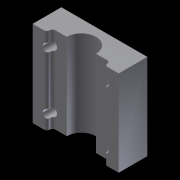
# Autodesk Inventor part: poleHolderA
Saved by Autodesk Inventor 2011 (Build 150239000, 239)
## iProperties
Created: 2012-10-15
Part Number: poleHolderA
Document SubType Name: Modeling
Designer: JohnHenry
Density: 1 g/cm^3
Author: JohnHenry
Autodesk Inventor part; units mm, degrees
ref_plane "YZ Plane" through (0, 0, 0) normal (1, 0, 0) x (0, 1, 0)
ref_plane "XZ Plane" through (0, 0, 0) normal (0, 1, 0) x (-1, 0, 0)
ref_plane "XY Plane" through (0, 0, 0) normal (0, 0, 1) x (1, 0, 0)
sketch "スケッチ1" plane through (0, 0, 0) normal (0, 0, 1) x (1, 0, 0)
  arc A0 (-5.1, 0) -> (5.1, 0) centre (0, 0) ccw
  line L0 (-15, 8) -> (15, 8)
  line L1 (15, 8) -> (15, 0)
  line L2 (15, 0) -> (5.1, 0)
  line L3 (-15, 0) -> (-15, 8)
  arc A1 (5.1, 0) -> (-5.1, 0) centre (0, 0) ccw
  line L4 (5.1, 0) -> (-5.1, 0)
  line L5 (-5.1, 0) -> (-15, 0)
  dimension "d0" = 10.2
  dimension "d1" = 30
  dimension "d2" = 15
  dimension "d3" = 8
  dimension "d4" = 0
  constraints: 12 end point, 4 parallel, 4 point on circle, 2 centre point, 1 coincident, 1 horizontal, 1 perpendicular, 1 point on line
  measures "d0" diameter of A0
  measures "d1" distance of L0.start L0.end
  measures "d2" distance from line of L3 point (0, 0)
  measures "d3" distance of L0.end L1.end
  measures "d4" distance from line of L2 point (0, 0)
extrude "押し出し1" add sketch "スケッチ1" along normal blind 30 contours L5 L3 L0 L1 L2 A1
sketch "スケッチ2" plane through (-15, 0, 0) normal (0, -1, 0) x (1, 0, 0)
  line L0 (9.9, 30) -> (0, 30) projected
  line L1 (0, 0) -> (9.9, 0) projected
  line L2 (0, 30) -> (4.95, 30)
  line L3 (4.95, 30) -> (4.95, 0)
  line L4 (4.95, 0) -> (0, 0)
  line L5 (0, 0) -> (0, 30)
  line L6 (30, 30) -> (25.05, 30)
  line L7 (25.05, 30) -> (25.05, 0)
  line L8 (25.05, 0) -> (30, 0)
  line L9 (30, 0) -> (30, 30)
  point P0 (15, 0)
  dimension "d7" = 30
  dimension "d8" = 4.95
  constraints: 16 end point, 4 parallel, 2 horizontal, 2 perpendicular, 1 midpoint, 1 point on line
  measures "d7" distance between parallel lines of L9 L5
  measures "d8" distance between parallel lines of L9 L7
extrude "押し出し2" add sketch "スケッチ2" along normal blind 2
fillet "フィレット1" radius 1 4 edges at (-10.05, -2, 15) (-10.05, 0, 15) (10.05, 0, 15) (10.05, -2, 15)
sketch "スケッチ3" plane through (-15, 8, 0) normal (0, 1, 0) x (1, 0, 0)
  line L0 (0, -30) -> (30, -30) projected
  line L1 (30, 0) -> (30, -30) projected
  line L2 (30, 0) -> (0, 0) projected
  line L3 (0, 0) -> (0, -30) projected
  point P0 (15, 0)
  point P1 (5, -5)
  point P2 (5, -25)
  point P3 (25, -25)
  point P4 (25, -5)
  dimension "d11" = 5
  dimension "d12" = 5
  dimension "d13" = 5
  dimension "d14" = 5
  dimension "d15" = 5
  dimension "d16" = 5
  dimension "d17" = 5
  dimension "d18" = 5
  measures "d11" distance from line of point (5, -5) L2
  measures "d12" distance from line of L3 point (5, -5)
  measures "d13" distance from line of L0 point (5, -25)
  measures "d14" distance from line of L3 point (5, -25)
  measures "d15" distance from line of L1 point (25, -25)
  measures "d16" distance from line of L0 point (25, -25)
  measures "d17" distance from line of L2 point (25, -5)
  measures "d18" distance from line of point (25, -5) L1
hole "Hole2" at (-10, 8, 5) at (-10, 8, 25) at (10, 8, 25) at (10, 8, 5) direction (0, -1, 0) diameter 3 end through all
equation "\"d2\" = 0.5 * d1"
equation "\"d12\" = d11"
equation "\"d13\" = d11"
equation "\"d14\" = d13"
equation "\"d15\" = d11"
equation "\"d16\" = d11"
equation "\"d17\" = d11"
equation "\"d18\" = d11"
